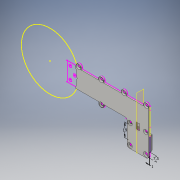
# Autodesk Inventor part: support_fourche_partie_capot
Saved by Autodesk Inventor 2016 (Build 200138000, 138)
## iProperties
Created: 2016-09-12
Part Number: support_fourche_partie_capot
Material: Generic
Document SubType Name: Modeling
Designer: mbouhier
Density: 1 g/cm^3
Appearance: Default
Author: mbouhier
Autodesk Inventor part; units mm, degrees
ref_plane "Work Plane1" through (0, 0, 0) normal (0, 0, 1) x (1, 0, 0)
ref_plane "Work Plane2" through (0, 0, 0) normal (0, 0, 1) x (1, 0, 0)
ref_plane "Work Plane3" through (0, 0, 0) normal (0, 0, 1) x (1, 0, 0)
ref_plane "Work Plane4" through (0, 0, 0) normal (0, 0, 1) x (1, 0, 0)
sketch "Sketch4" plane through (0, 0, 0) normal (0, 0, 1) x (1, 0, 0)
  line L0 (49.4972, -32.0028) -> (22.4972, -32.0028) projected
  line L1 (22.4972, -32.0028) -> (22.4972, -12.0028) projected
  line L2 (22.4972, -12.0028) -> (49.4972, -12.0028) projected
  line L3 (49.4972, -12.0028) -> (49.4972, -1.3028) projected
  line L4 (49.4972, -1.3028) -> (-34.5028, -1.3028) projected
  line L5 (-34.5028, -1.3028) -> (-34.5028, 19.2972) projected
  line L6 (-34.5028, 19.2972) -> (49.4972, 19.2972) projected
  line L7 (49.4972, 19.2972) -> (49.4972, 23.9972) projected
  arc A0 (49.4972, 23.9972) -> (42.4972, 23.9972) centre (45.9972, 23.9972) ccw projected
  line L8 (42.4972, 23.9972) -> (42.4972, 21.9972) projected
  line L9 (42.4972, 21.9972) -> (17.9972, 21.9972) projected
  line L10 (17.9972, 21.9972) -> (17.9972, 23.9972) projected
  arc A1 (17.9972, 23.9972) -> (10.9972, 23.9972) centre (14.4972, 23.9972) ccw projected
  line L11 (10.9972, 23.9972) -> (10.9972, 21.9972) projected
  line L12 (10.9972, 21.9972) -> (-13.5028, 21.9972) projected
  line L13 (-13.5028, 21.9972) -> (-13.5028, 23.9972) projected
  arc A2 (-13.5028, 23.9972) -> (-20.5028, 23.9972) centre (-17.0028, 23.9972) ccw projected
  line L14 (-20.5028, 23.9972) -> (-20.5028, 21.9972) projected
  line L15 (-20.5028, 21.9972) -> (-45.0028, 21.9972) projected
  line L16 (-45.0028, 21.9972) -> (-45.0028, 23.9972) projected
  arc A3 (-45.0028, 23.9972) -> (-52.0028, 23.9972) centre (-48.5028, 23.9972) ccw projected
  line L17 (-52.0028, 23.9972) -> (-52.0028, 21.9972) projected
  line L18 (-52.0028, 21.9972) -> (-66.5028, 21.9972) projected
  line L19 (-66.5028, 21.9972) -> (-66.5028, -4.0028) projected
  line L20 (-66.5028, -4.0028) -> (-20.0885, -4.0028) projected
  line L21 (-20.0885, -4.0028) -> (-20.0885, -6.0028) projected
  arc A4 (-20.0885, -6.0028) -> (-13.0885, -6.0028) centre (-16.5885, -6.0028) ccw projected
  line L22 (-13.0885, -6.0028) -> (-13.0885, -4.0028) projected
  line L23 (-13.0885, -4.0028) -> (16.4972, -4.0028) projected
  line L24 (19.4972, -7.0028) -> (19.4972, -36.0028) projected
  line L25 (22.4972, -39.0028) -> (46.4972, -39.0028) projected
  line L26 (49.4972, -36.0028) -> (49.4972, -32.0028) projected
  circle A5 centre (-48.5028, 23.9972) radius 2 projected
  circle A6 centre (-17.0028, 23.9972) radius 2 projected
  circle A7 centre (14.4972, 23.9972) radius 2 projected
  circle A8 centre (45.9972, 23.9972) radius 2 projected
  circle A9 centre (-16.5885, -6.0028) radius 2 projected
  circle A10 centre (45.4972, -8.0028) radius 2 projected
  circle A11 centre (23.4972, -35.0028) radius 2 projected
  circle A12 centre (45.4972, -35.0028) radius 2 projected
  circle A13 centre (23.4972, -8.0028) radius 2 projected
  circle A14 centre (-90.5028, 8.9972) radius 40 projected
  line L27 (49.4972, 19.2972) -> (49.4972, -1.3028) projected
  line L28 (49.4972, 19.2972) -> (-34.5028, 19.2972) projected
  line L29 (-34.5028, 19.2972) -> (-34.5028, -1.3028) projected
  line L30 (49.4972, -1.3028) -> (-34.5028, -1.3028) projected
  circle A15 centre (-90.5028, 8.9972) radius 40 projected
  line L31 (49.4972, -32.0028) -> (22.4972, -32.0028) projected
  line L32 (49.4972, -12.0028) -> (49.4972, -32.0028) projected
  line L33 (22.4972, -12.0028) -> (49.4972, -12.0028) projected
  line L34 (22.4972, -32.0028) -> (22.4972, -12.0028) projected
  arc A16 (19.4972, -36.0028) -> (22.4972, -39.0028) centre (22.4972, -36.0028) ccw projected
  arc A17 (46.4972, -39.0028) -> (49.4972, -36.0028) centre (46.4972, -36.0028) ccw projected
  arc A18 (19.4972, -7.0028) -> (16.4972, -4.0028) centre (16.4972, -7.0028) ccw projected
  circle A19 centre (-62.0028, 0.4972) radius 2 projected
  circle A20 centre (-62.0028, 17.4972) radius 2 projected
  circle A21 centre (-56.0028, 8.9972) radius 2 projected
  point P0 (0, 0)
extrude "Extrusion1" add sketch "Sketch4" along normal blind 2 contours L26 A17 L25 A16 L24 A18 L23 L22 A4 L21 L20 A14 L18 L17 A3 L16 L15 L14 A2 L13 L12 L11 A1 L10 L9 L8 A0 L7 L6 L5 L4 L3 L2 L1 L0 | L0 L1 L2 L32 | L4 L5 L6 L27 | L20 L19 L18 A14 | A5 | A6 | A7 | A8 | A9 | A10 | A11 | A12 | A13 | A19 | A20 | A21 picked at (-65.6501, 6.3234)
sketch "Sketch5" plane through (0, 0, 2) normal (0, 0, 1) x (1, 0, 0)
  circle A0 centre (-90.5028, 8.9972) radius 40 projected
  point P0 (0, 0)
extrude "Extrusion2" cut sketch "Sketch5" against normal blind 3
sketch "Sketch6" plane through (0, 0, 0) normal (0, 0, -1) x (-1, 0, 0)
  line L0 (-49.4972, -36.0028) -> (-49.4972, 23.9972) projected
  line L1 (-19.4972, -7.0028) -> (-19.4972, -36.0028) projected
  line L2 (13.0885, -4.0028) -> (-16.4972, -4.0028) projected
  line L3 (-22.4972, -39.0028) -> (-46.4972, -39.0028) projected
  line L4 (-49.4972, -31.5028) -> (-19.4972, -31.5028)
  line L5 (-19.4972, -31.5028) -> (-19.4972, -12.5028)
  line L6 (-19.4972, -12.5028) -> (-49.4972, -12.5028)
  line L7 (-49.4972, -12.5028) -> (-49.4972, -31.5028)
  line L8 (-49.4972, -31.5028) -> (-19.4972, -12.5028) construction
  line L9 (-19.4972, -31.5028) -> (-49.4972, -12.5028) construction
  line L10 (-19.4972, -7.0028) -> (-19.4972, -36.0028) projected
  line L11 (-49.4972, -36.0028) -> (-49.4972, 23.9972) projected
  line L12 (-48.4972, -12.5028) -> (-48.4972, -31.5028)
  point P0 (0, 0)
  point P1 (-19.4972, -21.5028)
  point P2 (-34.4972, -22.0028)
  dimension "d42" = 19
  dimension "d45" = 7.5
  dimension "d47" = 1
  constraints: 14 end point, 4 point on line, 3 midpoint, 3 perpendicular, 2 collinear, 2 parallel
  measures "d42" distance of L5.end L4.end
  measures "d45" distance between parallel lines of L4 L3
  measures "d47" distance between parallel lines of L0 L12
extrude "Extrusion3" add sketch "Sketch6" along normal blind 4.1
sketch "Sketch7" plane through (0, 0, 2) normal (0, 0, 1) x (1, 0, 0)
  circle A0 centre (-48.5028, 23.9972) radius 2 projected
  circle A1 centre (-17.0028, 23.9972) radius 2 projected
  circle A2 centre (14.4972, 23.9972) radius 2 projected
  circle A3 centre (45.9972, 23.9972) radius 2 projected
  circle A4 centre (-16.5885, -6.0028) radius 2 projected
  circle A5 centre (23.4972, -35.0028) radius 2 projected
  circle A6 centre (23.4972, -8.0028) radius 2 projected
  circle A7 centre (45.4972, -8.0028) radius 2 projected
  circle A8 centre (45.4972, -35.0028) radius 2 projected
  point P0 (0, 0)
hole "Hole1" at (-16.5885, -6.0028, 2) at (-17.0028, 23.9972, 2) at (-48.5028, 23.9972, 2) at (14.4972, 23.9972, 2) at (45.9972, 23.9972, 2) at (23.4972, -8.0028, 2) at (45.4972, -8.0028, 2) at (45.4972, -35.0028, 2) at (23.4972, -35.0028, 2) direction (0, 0, -1) diameter 3.5 end through all countersink diameter 6.3 countersink angle 90
ref_plane "Work Plane5" through (22.4972, -32.0028, -15) normal (1, 0, 0) x (0, 1, 0)
sketch "Sketch13" plane through (0, 0, 0) normal (0, 0, -1) x (-1, 0, 0)
  line L0 (-42.4972, 21.9972) -> (-17.9972, 21.9972) projected
  line L1 (-49.4972, -36.0028) -> (-49.4972, 23.9972) projected
  line L2 (-19.4972, -7.0028) -> (-19.4972, -36.0028) projected
  point P0 (0, 0)
  point P1 (-34.4972, -6.6528)
  point P2 (-49.4972, -12.0028)
  point P3 (-19.4972, -12.0028)
  dimension "d28" = 28.65
  dimension "d29" = 30
  dimension "d30" = 15
  measures "d28" distance from line of point (-34.497, -6.653) L0
  measures "d29" distance between parallel lines of L1 L2
  measures "d30" distance from line of point (-34.497, -6.653) L2
ref_plane "Work Plane6" through (34.4972, -6.6528, 0) normal (1, 0, 0) x (0, 0, -1)
sketch "Sketch14" plane through (34.4972, -6.6528, 0) normal (1, 0, 0) x (0, 0, -1)
  circle A0 centre (1.5, 0) radius 5.5
  line L0 (-2, -29.35) -> (-2, 30.65) construction
  circle A1 centre (1.5, 0) radius 5 construction
  line L1 (-3.5, 0) -> (-3.5, 4.6838) construction
  point P0 (0, 6.6528)
  point P1 (0, 0)
  dimension "d34" = 10
  dimension "d31" = 1.5
  dimension "d32" = 11
  constraints: 2 coincident, 2 end point, 1 centre point, 1 horizontal alignment, 1 vertical, 2 other
  measures "d31" distance of point (1.5, 0) point (0, 0)
  measures "d32" diameter of A0
extrude "Extrusion7" cut sketch "Sketch14" along normal mid plane 4.5
sketch "Sketch15" plane through (49.4972, -36.0028, 2) normal (1, 0, 0) x (0, 0, -1)
  line L0 (6.1, 4.5) -> (6.1, 23.5) projected
  line L1 (2, 4.5) -> (6.1, 4.5) projected
  line L2 (6.1, 23.5) -> (4.1, 23.5)
  line L3 (4.1, 23.5) -> (4.1, 4.5)
  line L4 (4.1, 4.5) -> (6.1, 4.5)
  line L5 (6.1, 4.5) -> (6.1, 23.5)
  point P0 (2, 36.0028)
  point P1 (6.1, 18.5)
  dimension "d48" = 2
  constraints: 8 end point, 2 parallel, 1 horizontal, 1 perpendicular, 1 point on line
  measures "d48" distance of L4.end L3.end
extrude "Extrusion8" cut sketch "Sketch15" against normal blind 1
equation "\"d30\" = 0.5 * d29"
body "Solid1"
